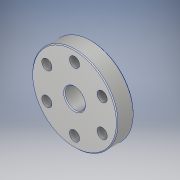
# Autodesk Inventor part: bepf_kolo_adapter_walu_fi6
Saved by Autodesk Inventor 2017 (Build 210142000, 142)
## iProperties
Created: 2016-11-23
Part Number: bepf_kolo_adapter_walu_fi6
Material: Aluminium 6061
Document SubType Name: Modeling
Designer: gagato
Density: 2.7 g/cm^3
Appearance: Aluminium — płaski
Mass: 6.83163 g
Surface Area: 18.4559 cm^2
Volume: 2.53023 cm^3
Author: gagato
Autodesk Inventor part; units mm, degrees
ref_plane "YZ Plane" through (0, 0, 0) normal (1, 0, 0) x (0, 1, 0)
ref_plane "XZ Plane" through (0, 0, 0) normal (0, 1, 0) x (-1, 0, 0)
ref_plane "XY Plane" through (0, 0, 0) normal (0, 0, 1) x (1, 0, 0)
sketch "Szkic1" plane through (0, 0, 0) normal (0, 0, 1) x (1, 0, 0)
  circle A0 centre (0, 0) radius 12.7
  dimension "d0" = 25.4
  constraints: 1 centre point, 1 coincident
  measures "d0" diameter of A0
extrude "Wyciągnięcie proste1" add sketch "Szkic1" along normal blind 4.2 and the other way blind 5
sketch "Szkic2" plane through (0, 0, 0) normal (0, 0, 1) x (1, 0, 0)
  circle A0 centre (0, 0) radius 6
  circle A1 centre (0, 0) radius 12.7 projected
  dimension "d5" = 12
  constraints: 1 centre point, 1 coincident
  measures "d5" diameter of A0
extrude "Wyciągnięcie proste2" cut sketch "Szkic2" along normal blind 4.2
hole "Otwór1" at (0, 0, 4.2) direction (0, 0, -1) diameter 6 end through all
sketch "Szkic3" plane through (0, 0, 0) normal (0, 0, 1) x (1, 0, 0)
  line L0 (0, 0) -> (0, 9.5) construction
  dimension "d18" = 9.5
  constraints: 2 end point, 1 coincident, 1 vertical
  measures "d18" distance of L0.start L0.end
hole "Otwór2" at (0, 9.5, 0) direction (0, 0, -1) diameter 3 end through all
pattern_circular "Szyk kołowy1" count 6 over 360 about axis through (0, 0, -32.8805) along (0, 0, 1) of "Otwór2"
chamfer "Faza1" distance 0.25 angle 45 6 edges at (-6, 0, 4.2) (-12.7, 0, 0) (-12.7, 0, -5) (-6, 0, 0) (0, 3, -5) (0, 3, 4.2)
move or copy body "Przesuń bryłę1" bodies to move or copy 1 copy no rotation origin (0, 0, 0) rotation axis (0, 1, 0) rotation angle 180
